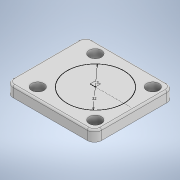
# Autodesk Inventor part: cylinder head
Saved by Autodesk Inventor 2020 (Build 240168000, 168)
## iProperties
Created: 2020-08-05
Part Number: cylinder head
Material: Generic
Document SubType Name: Modeling
Designer: benny
Density: 1 g/cm^3
Appearance: Default
Author: benny
Autodesk Inventor part; units mm, degrees
ref_plane "YZ Plane" through (0, 0, 0) normal (1, 0, 0) x (0, 1, 0)
ref_plane "XZ Plane" through (0, 0, 0) normal (0, 1, 0) x (-1, 0, 0)
ref_plane "XY Plane" through (0, 0, 0) normal (0, 0, 1) x (1, 0, 0)
sketch "Sketch1" plane through (0, 0, 0) normal (0, 1, 0) x (-1, 0, 0)
  line L0 (25, -22.5) -> (-25, -22.5)
  line L1 (-25, -22.5) -> (-25, 22.5)
  line L2 (-25, 22.5) -> (25, 22.5)
  line L3 (25, 22.5) -> (25, -22.5)
  line L4 (25, -22.5) -> (-25, 22.5) construction
  line L5 (-25, -22.5) -> (25, 22.5) construction
  line L6 (0, 0) -> (-3, 0)
  circle A0 centre (-3, 0) radius 16
  line L7 (-3, 0) -> (-19.2635, -16.2635)
  line L8 (-3, 0) -> (20, 0) construction
  circle A1 centre (-19.2635, -16.2635) radius 3.5
  dimension "d0" = 50
  dimension "d1" = 45
  dimension "d35" = 0
  dimension "d36" = 3
  dimension "d37" = 32
  dimension "d38" = 23
  dimension "d39" = 135
  dimension "d40" = 7
  constraints: 18 end point, 3 horizontal, 2 centre point, 2 coincident, 2 midpoint, 2 parallel, 1 equal length, 1 perpendicular
  measures "d0" distance of L1.end L2.end
  measures "d1" distance of L0.end L1.end
  measures "d35" distance of point (0, 0) L6.start
  measures "d36" distance of L6.start L6.end
  measures "d37" diameter of A0
  measures "d38" distance of L7.start L7.end
  measures "d39" angle of L7 L8
  measures "d40" diameter of A1
extrude "Extrusion1" add sketch "Sketch1" along normal blind 6 contours L0 L1 L2 L3 | A0 | A1
fillet "Fillet1" radius 4 4 edges at (25, 3, 22.5) (25, 3, -22.5) (-25, 3, -22.5) (-25, 3, 22.5)
fillet "Fillet2" radius 1 8 edges at (23.8284, 6, 21.3284) (25, 6, 0) (23.8284, 6, -21.3284) (0, 6, -22.5) (-23.8284, 6, -21.3284) (-25, 6, 0) (-23.8284, 6, 21.3284) (0, 6, 22.5)
sketch "Sketch6" plane through (0, 0, 0) normal (0, -1, 0) x (1, 0, 0)
  circle A0 centre (-3, -3) radius 18
  point P0 (0, 0)
  dimension "d21" = 36
  constraints: 1 centre point
  measures "d21" diameter of A0
extrude "Extrusion6" cut sketch "Sketch6" against normal blind 2
sketch "Sketch7" plane through (-3, 2, -3) normal (0, -1, 0) x (1, 0, 0)
  circle A0 centre (0, 0) radius 16
  point P0 (3, 3)
  dimension "d27" = 32
  constraints: 1 centre point
  measures "d27" diameter of A0
extrude "Extrusion7" add sketch "Sketch7" along normal blind 2
chamfer "Chamfer1" distance 1 distance2 1 1 edges at (-21, 0, -3) measured on face at (-21.5, 0, -3)
sketch "Sketch8" plane through (0, 6, 0) normal (0, 1, 0) x (1, 0, 0)
  line L0 (0, 0) -> (23, 0) construction
  constraints: 2 end point, 1 horizontal
sketch "Sketch9" plane through (0, 6, 0) normal (0, 1, 0) x (1, 0, 0)
  line L0 (0, 0) -> (3, 0)
  circle A0 centre (3, 0) radius 16
  dimension "d41" = 3
  dimension "d42" = 32
  constraints: 2 end point, 1 centre point, 1 coincident, 1 horizontal
  measures "d41" distance of L0.start L0.end
  measures "d42" diameter of A0
sketch "Sketch10" plane through (0, 6, 0) normal (0, 1, 0) x (1, 0, 0)
  line L0 (0, 0) -> (3, 0)
  line L1 (3, 0) -> (19.2635, 16.2635)
  circle A0 centre (19.2635, 16.2635) radius 3.5
  dimension "d43" = 3
  dimension "d44" = 23
  dimension "d45" = 135
  dimension "d46" = 7
  constraints: 4 end point, 1 centre point, 1 coincident, 1 horizontal
  measures "d43" distance of L0.start L0.end
  measures "d44" distance of L0.end L1.end
  measures "d45" angle of L1 L0
  measures "d46" diameter of A0
extrude "Extrusion8" cut sketch "Sketch10" against normal blind 10
sketch "Sketch11" plane through (0, 6, 0) normal (0, 1, 0) x (1, 0, 0)
  circle A0 centre (3, 0) radius 16
  point P0 (0, 0)
  dimension "d49" = 32
  constraints: 1 centre point
  measures "d49" diameter of A0
extrude "Extrusion9" cut sketch "Sketch11" against normal blind 2
pattern_circular "Circular Pattern2" count 4 over 360 about axis through (3, 6, 0) along (0, -1, 0) of "Extrusion8"
sketch "Sketch12" plane through (3, 4, 0) normal (0, 1, 0) x (1, 0, 0)
  circle A0 centre (0, 0) radius 16
  point P0 (-3, 0)
  dimension "d55" = 32
  constraints: 1 centre point
  measures "d55" diameter of A0
extrude "Extrusion10" add sketch "Sketch12" along normal blind 2
body "Solid1"
